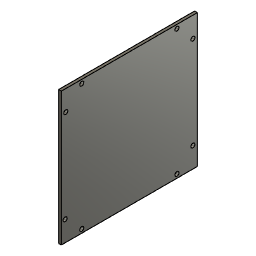
Боковые стенки Cubesat v16 (Autodesk Fusion 360 design; units mm, degrees)
Autodesk Fusion 360 part; units mm, degrees
note: some values were not read from the file. Set by a fixed rule: which sketch regions a step uses.
sketch "Sketch1" plane through (0, 0, 0) normal (1, 0, 0) x (0, 0, -1)
  line L0 (0, 0) -> (-100, 0)
  line L1 (-100, 0) -> (-100, 98)
  line L2 (-100, 98) -> (0, 98)
  line L3 (0, 98) -> (0, 0)
  dimension "d1" = 100
  dimension "d2" = 98
  constraint horizontal L0
  constraint vertical L1
  constraint horizontal L2
  constraint vertical L3
  constraint coincident L0.start L3.end
  measures "d1" distance of L0.start L0.end
  measures "d2" distance of L0.start L2.end
extrude "Extrude1" add sketch "Sketch1" against normal blind 2
extrude "Extrude2" add 1 faces at (0, 32.6667, 33.3333) along direction (1, 0, 0) blind 2
extrude "Extrude3" add 1 faces at (2, 32.6667, 33.3333) along direction (1, 0, 0) blind 1
sketch "Sketch2" plane through (3, 0, 0) normal (1, 0, 0) x (0, 0, -1)
  line L0 (-100, 98) -> (0, 98)
  line L1 (0, 98) -> (0, 0)
  line L2 (0, 0) -> (-100, 0)
  line L3 (-100, 0) -> (-100, 98)
  line L4 (-100, 98) -> (-85, 98)
  line L5 (-85, 98) -> (-85, 92.5)
  line L6 (-85, 92.5) -> (-100, 92.5)
  line L7 (-100, 92.5) -> (-100, 98)
  line L8 (-100, 98) -> (-93.5, 98)
  line L9 (-93.5, 98) -> (-93.5, 83)
  line L10 (0, 98) -> (-6.5, 98)
  line L11 (-6.5, 98) -> (-6.5, 83)
  line L12 (-6.5, 83) -> (0, 83)
  line L13 (0, 83) -> (0, 98)
  line L14 (0, 98) -> (-15, 98)
  line L15 (-15, 98) -> (-15, 92.5)
  line L16 (-15, 92.5) -> (0, 92.5)
  line L17 (0, 92.5) -> (0, 98)
  line L18 (0, 0) -> (-6.5, 0)
  line L19 (-6.5, 0) -> (-6.5, 15)
  line L20 (-6.5, 15) -> (0, 15)
  line L21 (0, 15) -> (0, 0)
  line L22 (0, 0) -> (-15, 0)
  line L23 (-15, 0) -> (-15, 5.5)
  line L24 (-15, 5.5) -> (0, 5.5)
  line L25 (0, 5.5) -> (0, 0)
  line L26 (-100, 0) -> (-85, 0)
  line L27 (-85, 0) -> (-85, 5.5)
  line L28 (-85, 5.5) -> (-100, 5.5)
  line L29 (-100, 5.5) -> (-100, 0)
  line L30 (-100, 0) -> (-94.5, 0)
  line L31 (-94.5, 0) -> (-94.5, 15)
  line L32 (-94.5, 15) -> (-100, 15)
  line L33 (-100, 15) -> (-100, 0)
  circle A0 centre (-85, 95.25) radius 1.5
  circle A1 centre (-97.25, 15) radius 1.5
  circle A2 centre (-85, 2.75) radius 1.5
  circle A3 centre (-15, 2.75) radius 1.5
  circle A4 centre (-3.25, 15) radius 1.5
  circle A5 centre (-3.25, 83) radius 1.5
  circle A6 centre (-15, 95.25) radius 1.5
  line L34 (-93.5, 83) -> (-100, 83)
  line L35 (-100, 83) -> (-100, 98)
  line L36 (-100, 98) -> (-93.5, 98)
  line L37 (-93.5, 98) -> (-93.5, 83)
  circle A7 centre (-96.75, 83) radius 1.5
  dimension "d53" = 15
  dimension "d54" = 5.5
  dimension "d55" = 6.5
  dimension "d57" = 6.5
  dimension "d58" = 15
  dimension "d59" = 15
  dimension "d60" = 5.5
  dimension "d61" = 6.5
  dimension "d62" = 15
  dimension "d63" = 5.5
  dimension "d64" = 15
  dimension "d65" = 5.5
  dimension "d66" = 15
  dimension "d67" = 100
  dimension "d68" = 98
  dimension "d69" = 5.5
  dimension "d70" = 15
  dimension "d71" = 3
  dimension "d73" = 3
  dimension "d74" = 3
  dimension "d75" = 3
  dimension "d76" = 3
  dimension "d77" = 3
  dimension "d78" = 3
  dimension "d81" = 15
  dimension "d83" = 3
  constraint horizontal L0
  constraint vertical L1
  constraint horizontal L2
  constraint vertical L3
  constraint coincident L1.end L2.start
  constraint horizontal L4
  constraint vertical L5
  constraint horizontal L6
  constraint vertical L7
  constraint horizontal L8
  constraint vertical L9
  constraint horizontal L10
  constraint vertical L11
  constraint horizontal L12
  constraint vertical L13
  constraint horizontal L14
  constraint vertical L15
  constraint horizontal L16
  constraint vertical L17
  constraint horizontal L18
  constraint vertical L19
  constraint horizontal L20
  constraint vertical L21
  constraint horizontal L22
  constraint vertical L23
  constraint horizontal L24
  constraint vertical L25
  constraint horizontal L26
  constraint vertical L27
  constraint horizontal L28
  constraint vertical L29
  constraint horizontal L30
  constraint vertical L31
  constraint horizontal L32
  constraint vertical L33
  constraint midpoint L5 A0.centre
  constraint midpoint L32 A1.centre
  constraint midpoint L27 A2.centre
  constraint midpoint L23 A3.centre
  constraint midpoint L20 A4.centre
  constraint midpoint L12 A5.centre
  constraint midpoint L15 A6.centre
  constraint horizontal L34
  constraint vertical L35
  constraint horizontal L36
  constraint vertical L37
  constraint midpoint L34 A7.centre
  measures "d53" distance of L0.start L4.end
  measures "d54" distance of L0.start L6.end
  measures "d55" distance of L0.start L8.end
  measures "d57" distance of L0.end L10.end
  measures "d58" distance of L0.end L12.end
  measures "d59" distance of L0.end L14.end
  measures "d60" distance of L0.end L16.end
  measures "d61" distance of L1.end L18.end
  measures "d62" distance of L1.end L20.end
  measures "d63" distance of L1.end L24.end
  measures "d64" distance of L2.end L26.end
  measures "d65" distance of L2.end L30.end
  measures "d66" distance of L2.end L32.end
  measures "d67" distance of L3 L13
  measures "d68" distance of L0 L2
  measures "d69" distance of L26 L28
  measures "d70" distance of L23 L25
  measures "d71" diameter of A0
  measures "d73" diameter of A1
  measures "d74" diameter of A2
  measures "d75" diameter of A3
  measures "d76" diameter of A4
  measures "d77" diameter of A5
  measures "d78" diameter of A6
  measures "d81" distance of L8 L34
  measures "d83" diameter of A7
extrude "Extrude9" cut sketch "Sketch2" against normal blind 20 contours L5 A0 | L5 A0 | L34 A7 | L34 A7 | L15 A6 | L15 A6 | L32 A1 | L32 A1 | L12 A5 | L12 A5 | L27 A2 | L27 A2 | L20 A4 | L20 A4 | L23 A3 | L23 A3
extrude "Extrude10" cut sketch "Sketch2" against normal blind 3 contours L0 L3 L4 L6 L7 L8 L9 L35 L36 L37 | L0 L4 L5 L6 L9 A0 L37 | L3 L6 L9 L34 L35 L37 A7 | L0 L1 L2 L3 L5 L6 L9 L11 L12 L15 L16 L19 L20 L23 L24 L27 L28 L31 L32 A0 A1 A2 A3 A4 A5 A6 L34 L37 A7 | L0 L11 L14 L15 L16 A6 | L3 L28 L31 L32 L33 A1 | L0 L1 L10 L11 L13 L14 L16 L17 | L2 L3 L26 L28 L29 L30 L31 L33 | L1 L11 L12 L13 L16 A5 | L2 L26 L27 L28 L31 A2 | L1 L19 L20 L21 L24 A4 | L2 L19 L22 L23 L24 A3 | L1 L2 L18 L19 L21 L22 L24 L25
